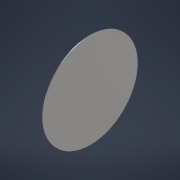
# Autodesk Inventor part: support disk-1
Saved by Autodesk Inventor 2021 (Build 250183000, 183)
## iProperties
Created: 2021-02-20
Part Number: support disk-1
Material: Steel, Mild
Document SubType Name: Modeling
Designer: vikki
Density: 7.85 g/cm^3
Appearance: Semi-Polished
Author: vikki
Autodesk Inventor part; units mm, degrees
ref_plane "YZ Plane" through (0, 0, 0) normal (1, 0, 0) x (0, 1, 0)
ref_plane "XZ Plane" through (0, 0, 0) normal (0, 1, 0) x (-1, 0, 0)
ref_plane "XY Plane" through (0, 0, 0) normal (0, 0, 1) x (1, 0, 0)
sketch "Sketch1" plane through (0, 0, 0) normal (1, 0, 0) x (0, 1, 0)
  circle A0 centre (0, 0) radius 136
  dimension "d0" = 272
  constraints: 1 centre point, 1 coincident
  measures "d0" diameter of A0
extrude "Extrusion1" add sketch "Sketch1" along normal blind 2
sketch "Sketch2" plane through (0, 0, 0) normal (-1, 0, 0) x (0, 0, 1)
  circle A0 centre (37.1481, 8.0013) radius 2.5 projected
  circle A1 centre (0, 0) radius 29 projected
  circle A2 centre (-37.1481, -8.0013) radius 2.5 projected
  circle A3 centre (-11.6447, -36.1718) radius 2.5 projected
  circle A4 centre (25.5034, -28.1705) radius 2.5 projected
  circle A5 centre (37.1481, 8.0013) radius 2.5 projected
  circle A6 centre (11.6447, 36.1718) radius 2.5 projected
  circle A7 centre (-25.5034, 28.1705) radius 2.5 projected
  circle A8 centre (40.2748, -102.3618) radius 4 projected
  circle A9 centre (-40.2748, 102.3618) radius 4 projected
  circle A10 centre (0, 0) radius 29 projected
  circle A11 centre (102.3618, 40.2748) radius 4 projected
  circle A12 centre (-102.3618, -40.2748) radius 4 projected
  circle A13 centre (0, 0) radius 135 projected
  point P0 (0, 0)
extrude "Extrusion2" cut sketch "Sketch2" against normal up to surface (2 mm away) contours A0 | A1 | A2 | A3 | A4 | A6 | A7 | A8 | A9 | A11 | A12
body "Solid1"
